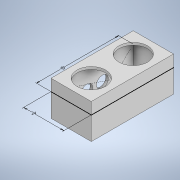
# Autodesk Inventor part: carcasaXeotype_ULTRASONIC
Saved by Autodesk Inventor 2020 (Build 240168000, 168)
## iProperties
Created: 2021-04-10
Part Number: carcasaXeotype_ULTRASONIC
Material: Generic
Document SubType Name: Modeling
Designer: Vlasciar
Density: 1 g/cm^3
Appearance: Default
Author: Vlasciar
Autodesk Inventor part; units mm, degrees
ref_plane "YZ Plane" through (0, 0, 0) normal (1, 0, 0) x (0, 1, 0)
ref_plane "XZ Plane" through (0, 0, 0) normal (0, 1, 0) x (-1, 0, 0)
ref_plane "XY Plane" through (0, 0, 0) normal (0, 0, 1) x (1, 0, 0)
sketch "Sketch1" plane through (0, 0, 0) normal (0, 1, 0) x (-1, 0, 0)
  line L0 (-12, -24.5) -> (12, -24.5)
  line L1 (12, -24.5) -> (12, 24.5)
  line L2 (12, 24.5) -> (-12, 24.5)
  line L3 (-12, 24.5) -> (-12, -24.5)
  line L4 (-12, -24.5) -> (12, 24.5) construction
  line L5 (12, -24.5) -> (-12, 24.5) construction
  point P0 (0, 0)
  dimension "d0" = 24
  dimension "d1" = 49
  constraints: 12 end point, 2 midpoint, 2 parallel, 1 horizontal, 1 perpendicular
  measures "d0" distance of L1.end L2.end
  measures "d1" distance of L0.end L1.end
extrude "Extrusion1" add sketch "Sketch1" along normal blind 5.4 and the other way blind 13.8
shell "Shell1" thickness 1.5 removed faces 1 at (4, 5.4, 8.1667)
sketch "Sketch2" plane through (-12, -13.8, 24.5) normal (-1, 0, 0) x (0, 0, 1)
  line L0 (0, 0) -> (0, 19.2) projected
  line L1 (-49, 19.2) -> (-49, 0) projected
  line L2 (0, 0) -> (-49, 0) projected
  line L3 (-49, 0) -> (-49, 19.2) projected
  line L4 (-49, 1.5) -> (0, 1.5)
  circle A0 centre (-29.15, 5) radius 3.5
  line L5 (-24.5, 13.8) -> (-24.5, 1.5)
  line L6 (-24.5, 11) -> (0, 11)
  line L7 (-24.5, 13) -> (-49, 13)
  circle A1 centre (-19.85, 5) radius 3.5
  point P0 (-24.5, 13.8)
  dimension "d7" = 1.5
  dimension "d8" = 3.5
  dimension "d9" = 7
  dimension "d10" = 4.65
  dimension "d11" = 7
  dimension "d12" = 1.15
  constraints: 8 end point, 5 point on line, 2 centre point, 2 perpendicular, 1 coincident, 1 horizontal, 1 midpoint, 1 parallel, 1 vertical
  measures "d7" distance between parallel lines of L2 L4
  measures "d8" distance from line of L4 point (-29.15, 5)
  measures "d9" diameter of A0
  measures "d10" distance from line of A0.centre L5
  measures "d11" diameter of A1
  measures "d12" distance edge to line of A1 L5
extrude "Extrusion2" cut sketch "Sketch2" against normal blind 5.4 contours A1 | A0
sketch "Sketch3" plane through (0, 5.4, 0) normal (0, 1, 0) x (1, 0, 0)
  line L0 (-10.5, 23) -> (10.5, 23) projected
  line L1 (10.5, 23) -> (10.5, -23) projected
  line L2 (10.5, -23) -> (-10.5, -23) projected
  line L3 (-12, 24.5) -> (-12, -24.5) projected
  line L4 (-12, -24.5) -> (12, -24.5) projected
  line L5 (12, -24.5) -> (12, 24.5) projected
  line L6 (12, 24.5) -> (-12, 24.5) projected
  line L7 (12, 24.5) -> (-12, 24.5)
  line L8 (-12, 24.5) -> (-12, -24.5)
  line L9 (-12, -24.5) -> (12, -24.5)
  line L10 (12, -24.5) -> (12, 24.5)
  circle A0 centre (0, 12.5) radius 8.5
  circle A1 centre (0, -12.5) radius 8.5
  point P0 (0, 0)
  dimension "d15" = 17
  dimension "d16" = 2
  dimension "d17" = 2
  dimension "d18" = 17
  dimension "d19" = 2
  dimension "d20" = 2
  constraints: 8 end point, 2 centre point, 2 parallel, 1 horizontal, 1 perpendicular
  measures "d15" diameter of A0
  measures "d16" distance edge to line of A0 L1
  measures "d17" distance edge to line of A0 L0
  measures "d18" diameter of A1
  measures "d19" distance edge to line of A1 L1
  measures "d20" distance edge to line of A1 L2
extrude "Extrusion3" add sketch "Sketch3" along normal blind 1.5
body "Solid1"
